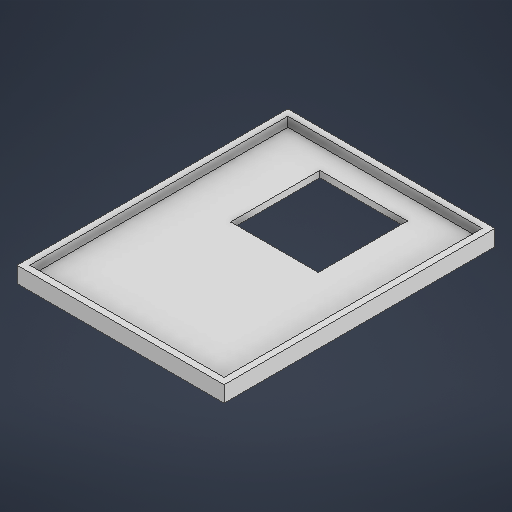
# Autodesk Inventor part: Tampa
Saved by Autodesk Inventor 2025 (Build 290162010, 162A)
## iProperties
Created: 2024-08-10
Part Number: Tampa
Material: Generic
Document SubType Name: Modeling
Designer: GabrielDBN
Density: 1 g/cm^3
Appearance: Default
Author: GabrielDBN
Autodesk Inventor part; units mm, degrees
ref_plane "YZ Plane" through (0, 0, 0) normal (1, 0, 0) x (0, 1, 0)
ref_plane "XZ Plane" through (0, 0, 0) normal (0, 1, 0) x (-1, 0, 0)
ref_plane "XY Plane" through (0, 0, 0) normal (0, 0, 1) x (1, 0, 0)
sketch "Sketch1" plane through (0, 0, 0) normal (0, 1, 0) x (-1, 0, 0)
  line L0 (30.8125, -40.4042) -> (-30.1875, -40.4042)
  line L1 (-30.1875, -40.4042) -> (-30.1875, 40.5958)
  line L2 (-30.1875, 40.5958) -> (30.8125, 40.5958)
  line L3 (30.8125, 40.5958) -> (30.8125, -40.4042)
  line L4 (-32.1875, -42.4042) -> (-32.1875, 42.5958)
  line L5 (32.8125, -42.4042) -> (-32.1875, -42.4042)
  line L6 (32.8125, -42.4042) -> (32.8125, 42.5958)
  line L7 (32.8125, 42.5958) -> (-32.1875, 42.5958)
  line L8 (14.0625, -33.7042) -> (-13.4375, -33.7042)
  line L9 (-13.4375, -33.7042) -> (-13.4375, -5.7042)
  line L10 (-13.4375, -5.7042) -> (14.0625, -5.7042)
  line L11 (14.0625, -5.7042) -> (14.0625, -33.7042)
  constraints: 24 end point, 4 perpendicular, 3 horizontal, 3 parallel, 2 vertical
extrude "Extrusion1" add sketch "Sketch1" along normal blind 2 contours L0 L1 L2 L3
extrude "Extrusion2" add sketch "Sketch1" along normal blind 5 contours L4 L7 L6 L5
body "Solid1"
